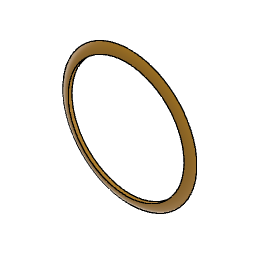
motor v23 (Autodesk Fusion 360 archive; units mm, degrees)
design "bottom ring"
Autodesk Fusion 360 part; units mm, degrees
sketch "Sketch1" plane through (0, 0, 0) normal (0, 0, 1) x (1, 0, 0)
  line L0 (0, 0) -> (80, 0)
  line L1 (80, 0) -> (80, 5)
  line L2 (80, 5) -> (92.5, 5)
  arc A0 (80, 0) -> (92.5, 5) centre (80, 18.125) ccw
  dimension "d2" = 80
  dimension "d3" = 5
  dimension "d4" = 12.5
  constraint coincident L0.start origin
  constraint horizontal L0
  constraint perpendicular L0 L1
  constraint perpendicular L1 L2
  constraint tangent L0 A0
  measures "d2" distance of L0.start L0.end
  measures "d3" distance of L0.end L1.end
  measures "d4" distance of L1.end L2.end
revolve "Revolve1" add sketch "Sketch1" angle 360 about axis through (0, 1.75, 0) along (0, 1, 0)

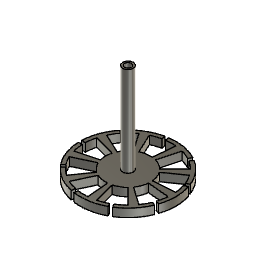
design "stator"
Autodesk Fusion 360 part; units mm, degrees
sketch "Sketch1" plane through (0, 0, 0) normal (0, 0, 1) x (1, 0, 0)
  circle A0 centre (0, 0) radius 7
  line L0 (0, 0) -> (64, 0) construction
  line L1 (56.1123, 18.232) -> (60.8676, 19.7771)
  line L2 (56.1123, -18.232) -> (60.8676, -19.7771)
  line L3 (0, 0) -> (64, 0) construction
  line L4 (29.8858, 2.6147) -> (58.7755, 5.1422)
  line L5 (29.8858, -2.6147) -> (58.7755, -5.1422)
  arc A1 (60.8676, -19.7771) -> (60.8676, 19.7771) centre (0, 0) ccw
  arc A2 (56.1123, -18.232) -> (58.7755, -5.1422) centre (0, 0) ccw
  arc A3 (58.7755, 5.1422) -> (56.1123, 18.232) centre (0, 0) ccw
  arc A4 (59.3398, 23.9748) -> (33.9148, 54.2751) centre (0, 0) ccw
  arc A5 (54.7038, 22.1018) -> (48.33, 33.841) centre (0, 0) ccw
  line L6 (54.7038, 22.1018) -> (59.3398, 23.9748)
  line L7 (31.2652, 50.0348) -> (33.9148, 54.2751)
  arc A6 (41.7193, 41.7193) -> (31.2652, 50.0348) centre (0, 0) ccw
  line L8 (21.2132, 21.2132) -> (41.7193, 41.7193)
  line L9 (24.5746, 17.2073) -> (48.33, 33.841)
  arc A7 (30.0462, 56.5086) -> (-8.9071, 63.3772) centre (0, 0) ccw
  arc A8 (27.6988, 52.0939) -> (15.2703, 56.9896) centre (0, 0) ccw
  line L10 (27.6988, 52.0939) -> (30.0462, 56.5086)
  line L11 (-8.2112, 58.4258) -> (-8.9071, 63.3772)
  arc A9 (5.1422, 58.7755) -> (-8.2112, 58.4258) centre (0, 0) ccw
  line L12 (2.6147, 29.8858) -> (5.1422, 58.7755)
  line L13 (7.7646, 28.9778) -> (15.2703, 56.9896)
  arc A10 (-13.3063, 62.6014) -> (-47.5613, 42.8244) centre (0, 0) ccw
  arc A11 (-12.2668, 57.7107) -> (-24.9345, 53.4722) centre (0, 0) ccw
  line L14 (-12.2668, 57.7107) -> (-13.3063, 62.6014)
  line L15 (-43.8455, 39.4787) -> (-47.5613, 42.8244)
  arc A12 (-33.841, 48.33) -> (-43.8455, 39.4787) centre (0, 0) ccw
  line L16 (-17.2073, 24.5746) -> (-33.841, 48.33)
  line L17 (-12.6785, 27.1892) -> (-24.9345, 53.4722)
  arc A13 (-50.4327, 39.4023) -> (-63.961, 2.2336) centre (0, 0) ccw
  arc A14 (-46.4926, 36.324) -> (-53.4722, 24.9345) centre (0, 0) ccw
  line L18 (-46.4926, 36.324) -> (-50.4327, 39.4023)
  line L19 (-58.9641, 2.0591) -> (-63.961, 2.2336)
  arc A15 (-56.9896, 15.2703) -> (-58.9641, 2.0591) centre (0, 0) ccw
  line L20 (-28.9778, 7.7646) -> (-56.9896, 15.2703)
  line L21 (-27.1892, 12.6785) -> (-53.4722, 24.9345)
  arc A16 (-63.961, -2.2336) -> (-50.4327, -39.4023) centre (0, 0) ccw
  arc A17 (-58.9641, -2.0591) -> (-56.9896, -15.2703) centre (0, 0) ccw
  line L22 (-58.9641, -2.0591) -> (-63.961, -2.2336)
  line L23 (-46.4926, -36.324) -> (-50.4327, -39.4023)
  arc A18 (-53.4722, -24.9345) -> (-46.4926, -36.324) centre (0, 0) ccw
  line L24 (-27.1892, -12.6785) -> (-53.4722, -24.9345)
  line L25 (-28.9778, -7.7646) -> (-56.9896, -15.2703)
  arc A19 (-47.5613, -42.8244) -> (-13.3063, -62.6014) centre (0, 0) ccw
  arc A20 (-43.8455, -39.4787) -> (-33.841, -48.33) centre (0, 0) ccw
  line L26 (-43.8455, -39.4787) -> (-47.5613, -42.8244)
  line L27 (-12.2668, -57.7107) -> (-13.3063, -62.6014)
  arc A21 (-24.9345, -53.4722) -> (-12.2668, -57.7107) centre (0, 0) ccw
  line L28 (-12.6785, -27.1892) -> (-24.9345, -53.4722)
  line L29 (-17.2073, -24.5746) -> (-33.841, -48.33)
  arc A22 (-8.9071, -63.3772) -> (30.0462, -56.5086) centre (0, 0) ccw
  arc A23 (-8.2112, -58.4258) -> (5.1422, -58.7755) centre (0, 0) ccw
  line L30 (-8.2112, -58.4258) -> (-8.9071, -63.3772)
  line L31 (27.6988, -52.0939) -> (30.0462, -56.5086)
  arc A24 (15.2703, -56.9896) -> (27.6988, -52.0939) centre (0, 0) ccw
  line L32 (7.7646, -28.9778) -> (15.2703, -56.9896)
  line L33 (2.6147, -29.8858) -> (5.1422, -58.7755)
  arc A25 (33.9148, -54.2751) -> (59.3398, -23.9748) centre (0, 0) ccw
  arc A26 (31.2652, -50.0348) -> (41.7193, -41.7193) centre (0, 0) ccw
  line L34 (31.2652, -50.0348) -> (33.9148, -54.2751)
  line L35 (54.7038, -22.1018) -> (59.3398, -23.9748)
  arc A27 (48.33, -33.841) -> (54.7038, -22.1018) centre (0, 0) ccw
  line L36 (24.5746, -17.2073) -> (48.33, -33.841)
  line L37 (21.2132, -21.2132) -> (41.7193, -41.7193)
  arc A28 (24.5746, -17.2073) -> (29.8858, -2.6147) centre (0, 0) ccw
  arc A29 (7.7646, -28.9778) -> (21.2132, -21.2132) centre (0, 0) ccw
  arc A30 (-12.6785, -27.1892) -> (2.6147, -29.8858) centre (0, 0) ccw
  arc A31 (-27.1892, -12.6785) -> (-17.2073, -24.5746) centre (0, 0) ccw
  arc A32 (-28.9778, 7.7646) -> (-28.9778, -7.7646) centre (0, 0) ccw
  arc A33 (-17.2073, 24.5746) -> (-27.1892, 12.6785) centre (0, 0) ccw
  arc A34 (2.6147, 29.8858) -> (-12.6785, 27.1892) centre (0, 0) ccw
  arc A35 (29.8858, 2.6147) -> (24.5746, 17.2073) centre (0, 0) ccw
  arc A36 (21.2132, 21.2132) -> (7.7646, 28.9778) centre (0, 0) ccw
  dimension "d1" = 128
  dimension "d2" = 14
  dimension "d3" = 60
  dimension "d6" = 64
  dimension "d10" = 360
  constraint coincident A0.centre L0.start
  constraint concentric A0 A1
  constraint concentric A1 A35
  constraint horizontal L0
  constraint symmetric L1.end L0 L2.end
  constraint symmetric L0 L1.start L2.start
  constraint horizontal L3
  constraint coincident L4.end A2
  constraint symmetric L3 L4.end L5.end
  constraint symmetric L3 L4.start L5.start
  constraint concentric A1 A2
  constraint concentric A2 A3
  constraint concentric A28 A35
  constraint concentric A29 A35
  constraint concentric A30 A35
  constraint concentric A31 A35
  constraint concentric A32 A35
  constraint concentric A33 A35
  constraint concentric A34 A35
  constraint concentric A35 A36
  measures "d1" diameter of A1
  measures "d2" diameter of A0
  measures "d3" diameter of A35
  measures "d6" distance of A0.centre L1.end
extrude "Extrude1" add sketch "Sketch1" along normal blind 11 makes body 1
sketch "Sketch2" plane through (0, 0, 11) normal (0, 0, 1) x (-1, 0, 0)
  circle A0 centre (0, 0) radius 7
  line L0 (-41.7193, -41.7193) -> (-21.2132, -21.2132)
  arc A1 (-21.2132, -21.2132) -> (-7.7646, -28.9778) centre (0, 0) ccw
  line L1 (-7.7646, -28.9778) -> (-15.2703, -56.9896)
  arc A2 (-27.6988, -52.0939) -> (-15.2703, -56.9896) centre (0, 0) ccw
  line L2 (-27.6988, -52.0939) -> (-30.0462, -56.5086)
  arc A3 (-30.0462, -56.5086) -> (8.9071, -63.3772) centre (0, 0) ccw
  line L3 (8.9071, -63.3772) -> (8.2112, -58.4258)
  arc A4 (-5.1422, -58.7755) -> (8.2112, -58.4258) centre (0, 0) ccw
  line L4 (-5.1422, -58.7755) -> (-2.6147, -29.8858)
  arc A5 (-2.6147, -29.8858) -> (12.6785, -27.1892) centre (0, 0) ccw
  line L5 (12.6785, -27.1892) -> (24.9345, -53.4722)
  arc A6 (12.2668, -57.7107) -> (24.9345, -53.4722) centre (0, 0) ccw
  line L6 (12.2668, -57.7107) -> (13.3063, -62.6014)
  arc A7 (13.3063, -62.6014) -> (47.5613, -42.8244) centre (0, 0) ccw
  line L7 (47.5613, -42.8244) -> (43.8455, -39.4787)
  arc A8 (33.841, -48.33) -> (43.8455, -39.4787) centre (0, 0) ccw
  line L8 (33.841, -48.33) -> (17.2073, -24.5746)
  arc A9 (17.2073, -24.5746) -> (27.1892, -12.6785) centre (0, 0) ccw
  line L9 (27.1892, -12.6785) -> (53.4722, -24.9345)
  arc A10 (46.4926, -36.324) -> (53.4722, -24.9345) centre (0, 0) ccw
  line L10 (46.4926, -36.324) -> (50.4327, -39.4023)
  arc A11 (50.4327, -39.4023) -> (63.961, -2.2336) centre (0, 0) ccw
  line L11 (63.961, -2.2336) -> (58.9641, -2.0591)
  arc A12 (56.9896, -15.2703) -> (58.9641, -2.0591) centre (0, 0) ccw
  line L12 (56.9896, -15.2703) -> (28.9778, -7.7646)
  arc A13 (28.9778, -7.7646) -> (28.9778, 7.7646) centre (0, 0) ccw
  line L13 (28.9778, 7.7646) -> (56.9896, 15.2703)
  arc A14 (58.9641, 2.0591) -> (56.9896, 15.2703) centre (0, 0) ccw
  line L14 (58.9641, 2.0591) -> (63.961, 2.2336)
  arc A15 (63.961, 2.2336) -> (50.4327, 39.4023) centre (0, 0) ccw
  line L15 (50.4327, 39.4023) -> (46.4926, 36.324)
  arc A16 (53.4722, 24.9345) -> (46.4926, 36.324) centre (0, 0) ccw
  line L16 (53.4722, 24.9345) -> (27.1892, 12.6785)
  arc A17 (27.1892, 12.6785) -> (17.2073, 24.5746) centre (0, 0) ccw
  line L17 (17.2073, 24.5746) -> (33.841, 48.33)
  arc A18 (43.8455, 39.4787) -> (33.841, 48.33) centre (0, 0) ccw
  line L18 (43.8455, 39.4787) -> (47.5613, 42.8244)
  arc A19 (47.5613, 42.8244) -> (13.3063, 62.6014) centre (0, 0) ccw
  line L19 (13.3063, 62.6014) -> (12.2668, 57.7107)
  arc A20 (24.9345, 53.4722) -> (12.2668, 57.7107) centre (0, 0) ccw
  line L20 (24.9345, 53.4722) -> (12.6785, 27.1892)
  arc A21 (12.6785, 27.1892) -> (-2.6147, 29.8858) centre (0, 0) ccw
  line L21 (-2.6147, 29.8858) -> (-5.1422, 58.7755)
  arc A22 (8.2112, 58.4258) -> (-5.1422, 58.7755) centre (0, 0) ccw
  line L22 (8.2112, 58.4258) -> (8.9071, 63.3772)
  arc A23 (8.9071, 63.3772) -> (-30.0462, 56.5086) centre (0, 0) ccw
  line L23 (-30.0462, 56.5086) -> (-27.6988, 52.0939)
  arc A24 (-15.2703, 56.9896) -> (-27.6988, 52.0939) centre (0, 0) ccw
  line L24 (-15.2703, 56.9896) -> (-7.7646, 28.9778)
  arc A25 (-7.7646, 28.9778) -> (-21.2132, 21.2132) centre (0, 0) ccw
  line L25 (-21.2132, 21.2132) -> (-41.7193, 41.7193)
  arc A26 (-31.2652, 50.0348) -> (-41.7193, 41.7193) centre (0, 0) ccw
  line L26 (-31.2652, 50.0348) -> (-33.9148, 54.2751)
  arc A27 (-33.9148, 54.2751) -> (-59.3398, 23.9748) centre (0, 0) ccw
  line L27 (-59.3398, 23.9748) -> (-54.7038, 22.1018)
  arc A28 (-48.33, 33.841) -> (-54.7038, 22.1018) centre (0, 0) ccw
  line L28 (-48.33, 33.841) -> (-24.5746, 17.2073)
  arc A29 (-24.5746, 17.2073) -> (-29.8858, 2.6147) centre (0, 0) ccw
  line L29 (-29.8858, 2.6147) -> (-58.7755, 5.1422)
  arc A30 (-56.1123, 18.232) -> (-58.7755, 5.1422) centre (0, 0) ccw
  line L30 (-56.1123, 18.232) -> (-60.8676, 19.7771)
  arc A31 (-60.8676, 19.7771) -> (-60.8676, -19.7771) centre (0, 0) ccw
  line L31 (-60.8676, -19.7771) -> (-56.1123, -18.232)
  arc A32 (-58.7755, -5.1422) -> (-56.1123, -18.232) centre (0, 0) ccw
  line L32 (-58.7755, -5.1422) -> (-29.8858, -2.6147)
  arc A33 (-29.8858, -2.6147) -> (-24.5746, -17.2073) centre (0, 0) ccw
  line L33 (-24.5746, -17.2073) -> (-48.33, -33.841)
  arc A34 (-54.7038, -22.1018) -> (-48.33, -33.841) centre (0, 0) ccw
  line L34 (-54.7038, -22.1018) -> (-59.3398, -23.9748)
  arc A35 (-59.3398, -23.9748) -> (-33.9148, -54.2751) centre (0, 0) ccw
  line L35 (-33.9148, -54.2751) -> (-31.2652, -50.0348)
  arc A36 (-41.7193, -41.7193) -> (-31.2652, -50.0348) centre (0, 0) ccw
  circle A37 centre (0, 0) radius 7
  constraint coincident A0.centre A1.centre
extrude "Extrude2" add sketch "Sketch2" along normal blind 120 separate body contours A0 A37 makes body 2
extrude "Extrude3" add 1 faces at (-1.3617, -1.5871, 11) along direction (0, 0, -1) blind 25 on bodies 2 bodies 2 1
sketch "Sketch3" plane through (0, 0, 131) normal (0, 0, 1) x (-1, 0, 0)
  circle A0 centre (0, 0) radius 7
  circle A1 centre (0, 0) radius 4.5
  dimension "d17" = 9
  constraint coincident A0.centre A1.centre
  measures "d17" diameter of A1
extrude "Extrude4" cut sketch "Sketch3" against normal through all contours A1 bodies 2

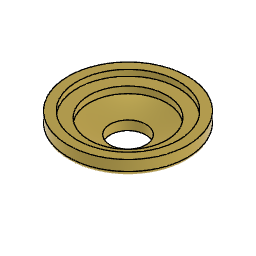
design "bottom"
Autodesk Fusion 360 part; units mm, degrees
sketch "Sketch1" plane through (0, 0, 0) normal (0, 1, 0) x (1, 0, 0)
  line L0 (30, 0) -> (80, 0)
  line L1 (80, 0) -> (80, -20)
  arc A0 (80, -20) -> (30, 0) centre (-12.0769, -177.6923) ccw
  line L2 (80, -20) -> (80, -25)
  line L3 (80, -25) -> (90, -25)
  line L4 (90, -25) -> (92.5, -25)
  line L5 (100, -32.5) -> (100, -50)
  arc A1 (100, -32.5) -> (92.5, -25) centre (92.5, -32.5) ccw
  line L6 (30, 0) -> (0, 0)
  line L7 (28.2102, -15) -> (0, -15)
  arc A2 (65, -28.8602) -> (28.2102, -15) centre (-12.0769, -177.6923) ccw
  line L8 (65, -28.8602) -> (65, -40)
  line L9 (65, -40) -> (85, -40)
  line L10 (85, -40) -> (85, -50)
  line L11 (85, -50) -> (100, -50)
  line L12 (0, -15) -> (0, 0)
  point P0 (100, -25)
  dimension "d2" = 30
  dimension "d3" = 50
  dimension "d4" = 20
  dimension "d5" = 5
  dimension "d6" = 10
  dimension "d7" = 10
  dimension "d8" = 25
  dimension "d9" = 7.5
  dimension "d15" = 30
  dimension "d17" = 182.6062
  dimension "d20" = 15
  constraint perpendicular L0 L1
  constraint parallel L1 L2
  constraint perpendicular L2 L3
  constraint parallel L3 L4
  constraint perpendicular L4 L5
  constraint coincident P0 L5
  constraint coincident P0 L4
  constraint tangent L5 A1
  constraint tangent L4 A1
  constraint coincident L6.end L12.end
  constraint parallel L0 L6
  constraint perpendicular L5 L11
  constraint perpendicular L6 L12
  measures "d2" distance of L6.end L0.start
  measures "d3" distance of L0.start L0.end
  measures "d4" distance of L0.end L1.end
  measures "d5" distance of L1.end L2.end
  measures "d6" distance of L2.end L3.end
  measures "d7" distance of L3.end P0
  measures "d8" distance of P0 L5.end
  measures "d9" radius of A1
  measures "d15" distance of L0.start L6.end
  measures "d17" radius of A0
revolve "Revolve1" add sketch "Sketch1" angle 360 about axis through (0, 0, 1.75) along (0, 0, 1) contours A0 L2 L3 L4 L5 A1 L6 L7 A2 L8 L9 L10 L11 L12
extrude "Extrude1" cut 1 faces at (12.4711, -5.3135, 15) along direction (0, 0, -1) blind 100
extrude "Extrude2" cut 1 faces at (29.2917, -1.4904, 0) along direction (0, 0, 1) through all
sketch "Sketch2" plane through (0, 0, 50) normal (0, 0, 1) x (-1, 0, 0)
  circle A0 centre (0, 0) radius 100
  circle A1 centre (0, 0) radius 85
  circle A2 centre (-92.5, 0) radius 2
  circle A3 centre (46.25, -80.1073) radius 2
  circle A4 centre (46.25, 80.1073) radius 2
  dimension "d25" = 4
  dimension "d27" = 360
  dimension "d27" = 360
  measures "d25" diameter of A2

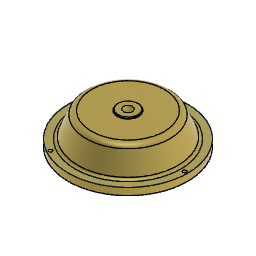
design "top half"
Autodesk Fusion 360 part; units mm, degrees
sketch "Sketch1" plane through (0, 0, 0) normal (0, 1, 0) x (1, 0, 0)
  line L0 (77.115, -50) -> (100, -50)
  line L1 (7.5, -91.0372) -> (7.5, -105)
  line L2 (7.5, -105) -> (16.5, -105)
  line L3 (17.5, -104) -> (17.5, -103.25)
  line L4 (17.75, -103) -> (60.8955, -103)
  line L5 (100, -50) -> (100, -62)
  line L6 (100, -62) -> (88.3023, -62)
  line L7 (70.0927, -96.9257) -> (83.7036, -65.0372)
  arc A0 (60.8955, -103) -> (70.0927, -96.9257) centre (60.8955, -93) ccw
  arc A1 (88.3023, -62) -> (83.7036, -65.0372) centre (88.3023, -67) ccw
  arc A2 (16.5, -105) -> (17.5, -104) centre (16.5, -104) ccw
  arc A3 (17.75, -103) -> (17.5, -103.25) centre (17.75, -103.25) ccw
  line L8 (56.2968, -91.0372) -> (69.9078, -59.1487)
  line L9 (56.2968, -91.0372) -> (7.5, -91.0372)
  line L10 (69.9078, -59.1487) -> (72.5164, -53.0372)
  arc A4 (77.115, -50) -> (72.5164, -53.0372) centre (77.115, -55) ccw
  point P0 (17.5, -105)
  point P1 (17.5, -103)
  point P2 (67.5, -103)
  point P3 (85, -62)
  dimension "d6" = 10
  dimension "d7" = 2
  dimension "d8" = 50
  dimension "d9" = 12
  dimension "d10" = 15
  dimension "d11" = 10
  dimension "d12" = 5
  dimension "d13" = 1
  dimension "d14" = 0.25
  dimension "d15" = -15
  dimension "d16" = 5
  dimension "d17" = 48.7968
  dimension "d18" = 13.9628
  constraint perpendicular L0 L1
  constraint perpendicular L1 L2
  constraint perpendicular L2 L3
  constraint perpendicular L3 L4
  constraint perpendicular L0 L5
  constraint perpendicular L5 L6
  constraint coincident P2 L4
  constraint coincident P2 L7
  constraint tangent L4 A0
  constraint tangent L7 A0
  constraint coincident P3 L7
  constraint coincident P3 L6
  constraint tangent L7 A1
  constraint tangent L6 A1
  constraint coincident P0 L2
  constraint coincident P0 L3
  constraint tangent L2 A2
  constraint tangent L3 A2
  constraint coincident P1 L3
  constraint coincident P1 L4
  constraint tangent L3 A3
  constraint tangent L4 A3
  constraint perpendicular L1 L9
  constraint parallel L8 L10
  constraint tangent L10 A4
  constraint tangent L0 A4
  measures "d6" distance of L1.end P0
  measures "d7" distance of P0 P1
  measures "d8" distance of P1 P2
  measures "d9" distance of L0.end L5.end
  measures "d10" distance of L5.end P3
  measures "d11" radius of A0
  measures "d12" radius of A1
  measures "d13" radius of A2
  measures "d14" radius of A3
  measures "d16" radius of A4
  measures "d17" distance of L8.start L1.start
  measures "d18" distance of L1.end L1.start
revolve "Revolve1" add sketch "Sketch1" angle 360 about axis through (0, 0, 1.75) along (0, 0, 1)
sketch "Sketch2" plane through (0, 0, 62) normal (0, 0, 1) x (-1, 0, 0)
  circle A0 centre (0, 0) radius 100
  circle A1 centre (0, 0) radius 88.3023
sketch "Sketch3" plane through (0, 0, 62) normal (0, 0, 1) x (1, 0, 0)
sketch "Sketch4" plane through (0, 0, 62) normal (0, 0, 1) x (-1, 0, 0)
  circle A0 centre (-95, 0) radius 3
  dimension "d22" = 6
  measures "d22" diameter of A0
extrude "Extrude1" cut sketch "Sketch4" against normal blind 8
pattern_circular "C-Pattern1" count 3 over 360 about axis through (0, 0, 1.75) along (0, 0, 1) of "Extrude1"

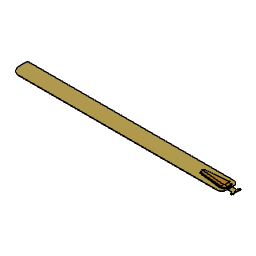
design "blade"
Autodesk Fusion 360 part; units mm, degrees
sketch "Sketch1" plane through (0, 0, 0) normal (0, 0, 1) x (1, 0, 0)
  line L0 (670, -55) -> (-645, -55)
  line L1 (-700, 0) -> (-700, 45)
  line L2 (-690, 55) -> (670, 55)
  line L3 (700, 25) -> (700, -25)
  line L4 (700, -55) -> (-700, 55) construction
  line L5 (-700, -55) -> (700, 55) construction
  arc A0 (-700, 0) -> (-645, -55) centre (-645, 0) ccw
  arc A1 (-690, 55) -> (-700, 45) centre (-690, 45) ccw
  arc A2 (700, 25) -> (670, 55) centre (670, 25) ccw
  arc A3 (670, -55) -> (700, -25) centre (670, -25) ccw
  dimension "d1" = 1400
  dimension "d2" = 110
  dimension "d3" = 55
  dimension "d4" = 10
  dimension "d5" = 30
  dimension "d6" = 30
  constraint horizontal L0
  constraint perpendicular L0 L1
  constraint parallel L0 L2
  constraint parallel L1 L3
  constraint coincident L4 origin
  constraint coincident L5 origin
  constraint coincident L5.start L1
  constraint coincident L5.start L0
  constraint tangent L1 A0
  constraint tangent L0 A0
  constraint coincident L4.end L2
  constraint coincident L4.end L1
  constraint tangent L2 A1
  constraint tangent L1 A1
  constraint coincident L5.end L2
  constraint coincident L5.end L3
  constraint tangent L2 A2
  constraint tangent L3 A2
  constraint coincident L4.start L0
  constraint coincident L4.start L3
  constraint tangent L0 A3
  constraint tangent L3 A3
  measures "d1" distance of L4.end L5.end
  measures "d2" distance of L5.start L4.end
  measures "d3" radius of A0
  measures "d4" radius of A1
  measures "d5" radius of A2
  measures "d6" radius of A3
surface "SurfacePatch1" add patch path "Sketch1" along A2 L3 A3 L0 A0 L1 A1 L2 makes body 1
form "Form1" [no effect]
thicken "Thicken1" add thickness 2 1 faces at (-221.6667, 18.3333, 0) separate body on bodies 1 makes body 2
sketch "Sketch4" plane through (0, 0, 0) normal (0, 0, -1) x (1, 0, 0)
  arc A0 (670, -55) -> (700, -25) centre (670, -25) ccw
  line L0 (700, -25) -> (700, 25)
  arc A1 (700, 25) -> (670, 55) centre (670, 25) ccw
  line L1 (670, 55) -> (-645, 55)
  arc A2 (-645, 55) -> (-700, 0) centre (-645, 0) ccw
  line L2 (-700, 0) -> (-700, -45)
  arc A3 (-700, -45) -> (-690, -55) centre (-690, -45) ccw
  line L3 (-690, -55) -> (670, -55)
  line L4 (675, 17.9402) -> (675, -17.9402)
  line L5 (658.0804, 32.8168) -> (535.2605, 16.9691)
  line L6 (520, -0.387) -> (520, 0.387)
  line L7 (535.2605, -16.9691) -> (658.0804, -32.8168)
  arc A4 (535.2605, 16.9691) -> (520, -0.387) centre (537.5, -0.387) ccw
  arc A5 (520, 0.387) -> (535.2605, -16.9691) centre (537.5, 0.387) ccw
  arc A6 (675, 17.9402) -> (658.0804, 32.8168) centre (660, 17.9402) ccw
  arc A7 (658.0804, -32.8168) -> (675, -17.9402) centre (660, -17.9402) ccw
  line L8 (675, 0) -> (675, 15)
  line L9 (675, 15) -> (721.7477, 15)
  line L10 (675, 0) -> (675, -15)
  line L11 (675, -15) -> (721.7477, -15)
  line L12 (738.4733, 32.7486) -> (743.8863, 29.2197)
  line L13 (1.75, 0) -> (22.5, 0)
  line L14 (738.4733, -32.7486) -> (743.8863, -29.2197)
  arc A8 (744.7402, 26.8224) -> (744.7402, -26.8224) centre (828.8358, 0) ccw
  arc A9 (733.8344, 31.1166) -> (731.4858, 22.7266) centre (828.8358, 0) ccw
  arc A10 (731.4858, -22.7266) -> (733.8344, -31.1166) centre (828.8358, 0) ccw
  arc A11 (738.4733, 32.7486) -> (733.8344, 31.1166) centre (736.7804, 30.1517) ccw
  arc A12 (744.7402, 26.8224) -> (743.8863, 29.2197) centre (742.7395, 27.4605) ccw
  arc A13 (733.8344, -31.1166) -> (738.4733, -32.7486) centre (736.7804, -30.1517) ccw
  arc A14 (743.8863, -29.2197) -> (744.7402, -26.8224) centre (742.7395, -27.4605) ccw
  arc A15 (731.4858, -22.7266) -> (721.7477, -15) centre (721.7477, -25) ccw
  arc A16 (721.7477, 15) -> (731.4858, 22.7266) centre (721.7477, 25) ccw
  point P0 (675, 35)
  point P1 (675, -35)
  point P2 (520, 15)
  point P3 (520, -15)
  point P4 (730, 15)
  point P5 (730, -15)
  dimension "d12" = 70
  dimension "d13" = 30
  dimension "d14" = 17.5
  dimension "d15" = 17.5
  dimension "d16" = 15
  dimension "d17" = 15
  dimension "d18" = 15
  dimension "d19" = 55
  dimension "d20" = 15
  dimension "d21" = 55
  dimension "d23" = 3.1
  dimension "d24" = 2.1
  dimension "d25" = 3.1
  dimension "d26" = 2.1
  dimension "d27" = 10
  dimension "d28" = 10
  constraint vertical L4
  constraint parallel L4 L6
  constraint coincident P2 L5
  constraint coincident P2 L6
  constraint tangent L5 A4
  constraint tangent L6 A4
  constraint coincident P3 L7
  constraint coincident P3 L6
  constraint tangent L7 A5
  constraint tangent L6 A5
  constraint coincident P0 L5
  constraint coincident P0 L4
  constraint tangent L5 A6
  constraint tangent L4 A6
  constraint coincident P1 L4
  constraint coincident P1 L7
  constraint tangent L4 A7
  constraint tangent L7 A7
  constraint midpoint L4 L8.start
  constraint parallel L4 L8
  constraint perpendicular L0 L9
  constraint parallel L4 L10
  constraint perpendicular L10 L11
  constraint coincident P5 A9
  constraint concentric A8 A9
  constraint concentric A9 A10
  constraint tangent A9 A11
  constraint tangent L12 A11
  constraint tangent L12 A12
  constraint tangent A8 A12
  constraint tangent A10 A13
  constraint tangent L14 A13
  constraint tangent A8 A14
  constraint tangent L14 A14
  constraint coincident P5 L11
  constraint coincident P5 A10
  constraint tangent L11 A15
  constraint tangent A10 A15
  constraint coincident P4 L9
  constraint coincident P4 A9
  constraint tangent L9 A16
  constraint tangent A9 A16
  measures "d12" distance of P0 P1
  measures "d13" distance of P2 P3
  measures "d14" radius of A4
  measures "d15" radius of A5
  measures "d16" radius of A6
  measures "d17" radius of A7
  measures "d18" distance of L8.start L8.end
  measures "d19" distance of L8.end P4
  measures "d20" distance of L8.start L10.end
  measures "d21" distance of L10.end P5
  measures "d23" radius of A11
  measures "d24" radius of A12
  measures "d25" radius of A13
  measures "d26" radius of A14
  measures "d27" radius of A15
  measures "d28" radius of A16
surface "SurfacePatch3" add patch profiles "Sketch4", "Sketch4", "Sketch4" section 1 contours L4 L5 L7 A4 A5 A6 A7 L8 L10 section 2 contours L0 L4 L8 L9 L10 L11 section 3 contours L0 L9 L11 L12 L14 A8 A9 A10 A11 A12 A13 A14 A15 A16 separate body makes body 3
thicken "Thicken3" add thickness 3 1 faces at (617.1405, 5.6564, 0) separate body on bodies 3 makes body 4
sketch "Sketch6" plane through (0, 0, 2) normal (0, 0, 1) x (-1, 0, 0)
  arc A0 (-700, -25) -> (-670, -55) centre (-670, -25) ccw
  line L0 (-670, -55) -> (690, -55)
  arc A1 (690, -55) -> (700, -45) centre (690, -45) ccw
  line L1 (700, -45) -> (700, 0)
  arc A2 (700, 0) -> (645, 55) centre (645, 0) ccw
  line L2 (645, 55) -> (-670, 55)
  arc A3 (-670, 55) -> (-700, 25) centre (-670, 25) ccw
  line L3 (-700, 25) -> (-700, -25)
  line L4 (-690, 0) -> (-690, -13.6304)
  line L5 (-690, 0) -> (-690, 13.6304)
  line L6 (-673.6927, -28.5733) -> (-524.3776, -15.5099)
  line L7 (-690, -30) -> (-510, -30) construction
  line L8 (-673.6927, 28.5733) -> (-524.3776, 15.5099)
  line L9 (-690, 30) -> (-510, 30) construction
  line L10 (-510.685, 0.567) -> (-510.685, -0.567)
  arc A4 (-524.3776, -15.5099) -> (-510.685, -0.567) centre (-525.685, -0.567) ccw
  arc A5 (-510.685, 0.567) -> (-524.3776, 15.5099) centre (-525.685, 0.567) ccw
  arc A6 (-690, -13.6304) -> (-673.6927, -28.5733) centre (-675, -13.6304) ccw
  arc A7 (-673.6927, 28.5733) -> (-690, 13.6304) centre (-675, 13.6304) ccw
  point P0 (-510.685, -14.312)
  point P1 (-510.685, 14.312)
  dimension "d30" = 30
  dimension "d31" = 30
  dimension "d32" = 180
  dimension "d33" = 5
  dimension "d34" = 180
  dimension "d35" = 5
  dimension "d36" = 15
  dimension "d37" = 15
  dimension "d38" = 15
  dimension "d39" = 15
  constraint vertical L4
  constraint parallel L4 L5
  constraint horizontal L7
  constraint horizontal L9
  constraint coincident P0 L6
  constraint coincident P0 L10
  constraint tangent L6 A4
  constraint tangent L10 A4
  constraint coincident P1 L10
  constraint coincident P1 L8
  constraint tangent L10 A5
  constraint tangent L8 A5
  constraint coincident L7.start L6
  constraint coincident L7.start L4
  constraint tangent L6 A6
  constraint tangent L4 A6
  constraint coincident L9.start L5
  constraint coincident L9.start L8
  constraint tangent L5 A7
  constraint tangent L8 A7
  measures "d30" distance of L4.start L7.start
  measures "d31" distance of L4.start L9.start
  measures "d32" distance of L7.start P0
  measures "d33" angle of L6 L7
  measures "d34" distance of L9.start P1
  measures "d35" angle of L8 L9
  measures "d36" radius of A4
  measures "d37" radius of A5
  measures "d38" radius of A6
  measures "d39" radius of A7
surface "SurfacePatch4" add patch path "Sketch6" along L10 A5 L8 A7 L5 L4 A6 L6 A4 separate body makes body 5
extrude "Extrude1" add 1 faces at (623.921, 5.17, 2) along direction (0, 0, 1) blind 15 draft -5 on bodies 5 bodies 2
fillet "Fillet1" radius 10 8 edges at (688.6877, 0, 17) (684.2473, -23.722, 17) (599.1495, -20.7343, 17) (515.5933, -9.8143, 17) (511.9973, 0, 17) (515.5933, 9.8143, 17) (599.1495, 20.7343, 17) (684.2473, 23.722, 17) on bodies 2
fillet "Fillet2" radius 3 8 edges at (510.685, 0, 2) (514.6258, 10.7009, 2) (599.0351, 22.0416, 2) (685.1339, 24.6895, 2) (690, 0, 2) (685.1339, -24.6895, 2) (599.0351, -22.0416, 2) (514.6258, -10.7009, 2) on bodies 2
split "Split1" by plane through (0.5668, 0.4592, 2) normal (0, 0, 1) bodies 2 makes body 6 at (624.834, 1.6914, 17)
sketch "Sketch7" plane through (0, 0, -3) normal (0, 0, -1) x (1, 0, 0)
  arc A0 (675, 17.9402) -> (658.0804, 32.8168) centre (660, 17.9402) ccw
  line L0 (658.0804, 32.8168) -> (535.2605, 16.9691)
  arc A1 (535.2605, 16.9691) -> (520.0043, 0) centre (537.5, -0.387) ccw
  arc A2 (520.0043, 0) -> (535.2605, -16.9691) centre (537.5, 0.387) ccw
  line L1 (535.2605, -16.9691) -> (658.0804, -32.8168)
  arc A3 (658.0804, -32.8168) -> (675, -17.9402) centre (660, -17.9402) ccw
  line L2 (675, -17.9402) -> (675, -15)
  line L3 (675, -15) -> (721.7477, -15)
  arc A4 (731.4858, -22.7266) -> (721.7477, -15) centre (721.7477, -25) ccw
  arc A5 (731.4858, -22.7266) -> (733.8344, -31.1166) centre (828.8358, 0) ccw
  arc A6 (733.8344, -31.1166) -> (738.4733, -32.7486) centre (736.7804, -30.1517) ccw
  line L4 (738.4733, -32.7486) -> (743.8863, -29.2197)
  arc A7 (743.8863, -29.2197) -> (744.7402, -26.8224) centre (742.7395, -27.4605) ccw
  arc A8 (744.7402, 26.8224) -> (744.7402, -26.8224) centre (828.8358, 0) ccw
  arc A9 (744.7402, 26.8224) -> (743.8863, 29.2197) centre (742.7395, 27.4605) ccw
  line L5 (743.8863, 29.2197) -> (738.4733, 32.7486)
  arc A10 (738.4733, 32.7486) -> (733.8344, 31.1166) centre (736.7804, 30.1517) ccw
  arc A11 (733.8344, 31.1166) -> (731.4858, 22.7266) centre (828.8358, 0) ccw
  arc A12 (721.7477, 15) -> (731.4858, 22.7266) centre (721.7477, 25) ccw
  line L6 (721.7477, 15) -> (675, 15)
  line L7 (675, 15) -> (675, 17.9402)
  circle A13 centre (735, 0) radius 3
  dimension "d46" = 6
  measures "d46" diameter of A13
extrude "Extrude2" cut sketch "Sketch7" against normal blind 12 contours A13 bodies 4
sketch "Sketch8" plane through (0, 0, -3) normal (0, 0, -1) x (1, 0, 0)
  circle A0 centre (735, 0) radius 3
  arc A1 (675, 17.9402) -> (658.0804, 32.8168) centre (660, 17.9402) ccw
  line L0 (658.0804, 32.8168) -> (535.2605, 16.9691)
  arc A2 (535.2605, 16.9691) -> (520.0043, 0) centre (537.5, -0.387) ccw
  arc A3 (520.0043, 0) -> (535.2605, -16.9691) centre (537.5, 0.387) ccw
  line L1 (535.2605, -16.9691) -> (658.0804, -32.8168)
  arc A4 (658.0804, -32.8168) -> (675, -17.9402) centre (660, -17.9402) ccw
  line L2 (675, -17.9402) -> (675, -15)
  line L3 (675, -15) -> (721.7477, -15)
  arc A5 (731.4858, -22.7266) -> (721.7477, -15) centre (721.7477, -25) ccw
  arc A6 (731.4858, -22.7266) -> (733.8344, -31.1166) centre (828.8358, 0) ccw
  arc A7 (733.8344, -31.1166) -> (738.4733, -32.7486) centre (736.7804, -30.1517) ccw
  line L4 (738.4733, -32.7486) -> (743.8863, -29.2197)
  arc A8 (743.8863, -29.2197) -> (744.7402, -26.8224) centre (742.7395, -27.4605) ccw
  arc A9 (744.7402, 26.8224) -> (744.7402, -26.8224) centre (828.8358, 0) ccw
  arc A10 (744.7402, 26.8224) -> (743.8863, 29.2197) centre (742.7395, 27.4605) ccw
  line L5 (743.8863, 29.2197) -> (738.4733, 32.7486)
  arc A11 (738.4733, 32.7486) -> (733.8344, 31.1166) centre (736.7804, 30.1517) ccw
  arc A12 (733.8344, 31.1166) -> (731.4858, 22.7266) centre (828.8358, 0) ccw
  arc A13 (721.7477, 15) -> (731.4858, 22.7266) centre (721.7477, 25) ccw
  line L6 (721.7477, 15) -> (675, 15)
  line L7 (675, 15) -> (675, 17.9402)
  circle A14 centre (737, 24) radius 2
  line L8 (1.75, 0) -> (22.5, 0)
  circle A15 centre (737, -24) radius 2
  dimension "d49" = 4
  constraint symmetric A14 L8 A15
  measures "d49" diameter of A14
extrude "Extrude3" cut sketch "Sketch8" against normal blind 7 contours A14 | A15 bodies 4
hidden bodies 1 3

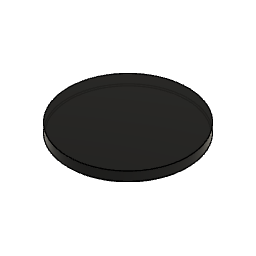
design "bottomglass"
Autodesk Fusion 360 part; units mm, degrees
sketch "Sketch1" plane through (0, 0, 0) normal (0, 0, 1) x (1, 0, 0)
  circle A0 centre (0, 0) radius 30
  dimension "d1" = 60
  constraint coincident A0.centre origin
  measures "d1" diameter of A0
extrude "Extrude1" add sketch "Sketch1" along normal blind 5
fillet "Fillet1" radius 0.5 1 edges at (-27.9698, -10.8485, 0)
